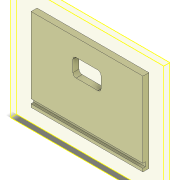
# Autodesk Inventor part: Lidar Sensor Case 4 v2 CNC
Saved by Autodesk Inventor 2018.3 (Build 223284000, 284)
## iProperties
Created: 2019-05-06
Part Number: Lidar Sensor Case 4 v2 CNC
Material: Generic
Document SubType Name: Modeling
Designer: aye06091
Mass: 6.36624 g
Surface Area: 51.9068 cm^2
Volume: 6.36624 cm^3
Density: 1 g/cm^3
Appearance: Default
Author: aye06091
Autodesk Inventor part; units mm, degrees
ref_plane "YZ Plane" through (0, 0, 0) normal (1, 0, 0) x (0, 1, 0)
ref_plane "XZ Plane" through (0, 0, 0) normal (0, 1, 0) x (-1, 0, 0)
ref_plane "XY Plane" through (0, 0, 0) normal (0, 0, 1) x (1, 0, 0)
sketch "Sketch1" plane through (0, 0, 0) normal (0, 0, 1) x (1, 0, 0)
  line L0 (0, 0) -> (55.626, 0)
  line L1 (55.626, 0) -> (55.626, -41.275)
  line L2 (55.626, -41.275) -> (0, -41.275)
  line L3 (0, -41.275) -> (0, 0)
  dimension "d0" = 41.275
  dimension "d1" = 55.626
  constraints: 8 end point, 2 parallel, 1 horizontal, 1 perpendicular
  measures "d0" distance of L2.end L0.start
  measures "d1" distance of L0.start L0.end
extrude "Extrusion1" add sketch "Sketch1" against normal blind 2.9972
sketch "Sketch2" plane through (0, 0, 0) normal (0, 0, 1) x (1, 0, 0)
  line L0 (0, -41.275) -> (0, 0) projected
  line L1 (55.626, -41.275) -> (0, -41.275) projected
  line L2 (20.828, -8.5598) -> (34.798, -8.5598)
  line L3 (34.798, -8.5598) -> (34.798, -17.4498)
  line L4 (34.798, -17.4498) -> (20.828, -17.4498)
  line L5 (20.828, -17.4498) -> (20.828, -8.5598)
  dimension "d4" = 13.97
  dimension "d5" = 8.89
  dimension "d6" = 20.828
  dimension "d7" = 23.8252
  constraints: 8 end point, 2 parallel, 1 horizontal, 1 perpendicular
  measures "d4" distance of L2.start L2.end
  measures "d5" distance of L4.end L2.start
  measures "d6" distance between parallel lines of L0 L5
  measures "d7" distance between parallel lines of L1 L4
extrude "Extrusion2" cut sketch "Sketch2" against normal blind 2.9972
fillet "Fillet1" radius 1.5875 4 edges at (20.828, -17.4498, -1.4986) (20.828, -8.5598, -1.4986) (34.798, -8.5598, -1.4986) (34.798, -17.4498, -1.4986)
sketch "Sketch3" plane through (0, 0, 0) normal (0, 0, 1) x (1, 0, 0)
  line L0 (0, -41.275) -> (0, 0) projected
  line L1 (55.626, -41.275) -> (0, -41.275) projected
  line L2 (55.626, 0) -> (55.626, -41.275) projected
  line L3 (0, -39.6875) -> (55.626, -39.6875)
  line L4 (55.626, -39.6875) -> (55.626, -37.5285)
  line L5 (55.626, -37.5285) -> (0, -37.5285)
  line L6 (0, -37.5285) -> (0, -39.6875)
  dimension "d11" = 1.5875
  dimension "d12" = 2.159
  constraints: 8 end point, 2 parallel, 2 point on line, 1 horizontal, 1 perpendicular
  measures "d11" distance between parallel lines of L1 L3
  measures "d12" distance between parallel lines of L3 L5
extrude "Extrusion3" cut sketch "Sketch3" against normal blind 1.2446 contours L0 L5 L2 L3
body "Solid1"
